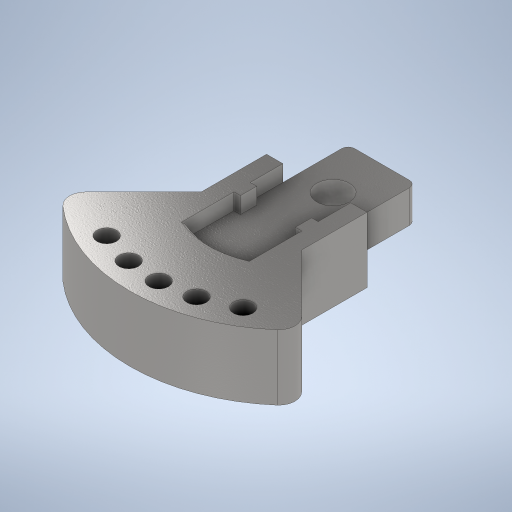
# Autodesk Inventor part: werkzeug
Saved by Autodesk Inventor 2024 (Build 280153000, 153)
## iProperties
Created: 2024-02-08
Part Number: werkzeug
Material: Stahl, galvanisiert
Document SubType Name: Modeling
Designer: ffogue
Density: 7.85 g/cm^3
Appearance: Galvanisiert
Author: ffogue
Autodesk Inventor part; units mm, degrees
ref_plane "YZ Plane" through (0, 0, 0) normal (1, 0, 0) x (0, 1, 0)
ref_plane "XZ Plane" through (0, 0, 0) normal (0, 1, 0) x (-1, 0, 0)
ref_plane "XY Plane" through (0, 0, 0) normal (0, 0, 1) x (1, 0, 0)
sketch "Skizze1" plane through (0, 0, 0) normal (0, 0, 1) x (1, 0, 0)
  line L0 (19.1421, 31.2132) -> (19.1421, 61.2132)
  line L1 (19.1421, 61.2132) -> (39.9308, 61.2132)
  line L2 (39.9308, 61.2132) -> (39.9308, 31.2132)
  line L3 (39.9308, 31.2132) -> (37.9308, 31.2132)
  line L4 (37.9308, 31.2132) -> (37.9308, 26.2132)
  line L5 (37.9308, 26.2132) -> (39.9308, 26.2132)
  line L6 (39.9308, 26.2132) -> (39.9308, 11.2132)
  line L7 (19.1421, 31.2132) -> (21.1421, 31.2132)
  line L8 (21.1421, 31.2132) -> (21.1421, 26.2132)
  line L9 (21.1421, 26.2132) -> (19.1421, 26.2132)
  line L10 (19.1421, 26.2132) -> (19.1421, 11.2132)
  line L11 (39.9308, 41.2132) -> (44.9308, 41.2132)
  line L12 (44.9308, 41.2132) -> (44.9308, 21.2132)
  line L13 (19.1421, 41.2132) -> (14.1421, 41.2132)
  line L14 (14.1421, 41.2132) -> (14.1421, 21.2132)
  line L15 (14.1421, 21.2132) -> (-3.5355, 3.5355)
  arc A0 (-3.5355, 3.5355) -> (-3.2818, -3.7722) centre (0, 0) ccw
  line L16 (44.9308, 21.2132) -> (62.6085, 3.5355)
  arc A1 (62.3548, -3.7722) -> (62.6085, 3.5355) centre (59.073, 0) ccw
  arc A2 (-3.2818, -3.7722) -> (62.3548, -3.7722) centre (29.5365, 33.9499) ccw
  arc A3 (19.1421, 11.2132) -> (39.9308, 11.2132) centre (29.5365, 33.9499) ccw
  line L17 (29.5365, 33.9499) -> (29.5365, 10.2757) construction
  dimension "d0" = 90
  dimension "d1" = 5
  dimension "d2" = 50
  dimension "d3" = 25
  dimension "d4" = 20
  dimension "d5" = 10
  dimension "d6" = 5
  dimension "d7" = 5
  dimension "d8" = 30
  dimension "d9" = 2
  dimension "d10" = 15
  dimension "d11" = 25
  constraints: 36 end point, 11 perpendicular, 8 point on circle, 7 point on line, 4 centre point, 4 horizontal alignment, 4 tangent, 2 horizontal, 2 vertical, 1 coincident, 1 concentric, 1 equal radius, 4 other
  measures "d0" angle of L15 L16
  measures "d1" radius of A0
  measures "d2" radius of A2
  measures "d3" radius of A3
  measures "d4" distance from line of L14.end L13
  measures "d5" distance between parallel lines of L11 L3
  measures "d6" distance from line of L4.end L3
  measures "d7" distance between parallel lines of L0 L14
  measures "d8" distance between parallel lines of L7 L1
  measures "d9" distance between parallel lines of L0 L8
  measures "d10" distance from line of L10.end L9
  measures "d11" distance of L14.end L15.end
extrude "Extrusion1" add sketch "Skizze1" along normal mid plane 10 contours L0 L1 L2 L3 L4 L5 L6 A3 L10 L9 L8 L7
extrude "Extrusion2" add sketch "Skizze1" along normal mid plane 20 contours L7 L8 L9 L10 A3 L6 L5 L4 L3 L2 L11 L12 L16 A1 A2 A0 L15 L14 L13 L0
sketch "Skizze2" plane through (0, 0, 5) normal (0, 0, 1) x (1, 0, 0)
  line L0 (39.9308, 61.2132) -> (19.1421, 61.2132) projected
  line L1 (29.5365, 61.2132) -> (29.5365, 18.1861) construction
  point P0 (0, 0)
  point P1 (29.5365, 46.2132)
  dimension "d16" = 15
  constraints: 2 end point, 1 midpoint, 1 point on line, 1 vertical
  measures "d16" distance from line of L0 point (29.536, 46.213)
hole "Bohrung1" at (29.5365, 46.2132, 5) direction (0, 0, -1) diameter 10 depth 10
chamfer "Fasen1" distance 1 angle 45 2 edges at (29.5365, 8.9499, 10) (29.5365, 8.9499, -10)
sketch "Skizze3" plane through (0, 0, 10) normal (0, 0, 1) x (1, 0, 0)
  arc A0 (6.4055, -2.2397) -> (53.6752, -1.5754) centre (29.5365, 33.9499) ccw construction
  arc A1 (-3.2818, -3.7722) -> (62.3548, -3.7722) centre (29.5365, 33.9499) ccw projected
  point P0 (0, 0)
  point P1 (21.3005, -8.2034)
  point P2 (31.2715, -8.9654)
  point P3 (41.2715, -7.3662)
  point P4 (51.2715, -3.0949)
  point P5 (11.3005, -4.9369)
  dimension "d27" = 10
  dimension "d28" = 10
  dimension "d29" = 10
  dimension "d30" = 10
  constraints: 7 point on circle, 1 centre point, 1 concentric
  measures "d27" distance of point (31.271, -8.965) point (21.301, -8.203)
  measures "d28" horizontal distance of point (41.271, -7.366) point (31.271, -8.965)
  measures "d29" horizontal distance of point (21.301, -8.203) point (11.301, -4.937)
  measures "d30" horizontal distance of point (51.271, -3.095) point (41.271, -7.366)
hole "Bohrung2" at (21.3005, -8.2034, 10) at (31.2715, -8.9654, 10) at (41.2715, -7.3662, 10) at (51.2715, -3.0949, 10) at (11.3005, -4.9369, 10) direction (0, 0, -1) diameter 6 end through all
fillet "Rundung1" radius 2 2 edges at (19.1421, 61.2132, 0) (39.9308, 61.2132, 0)
